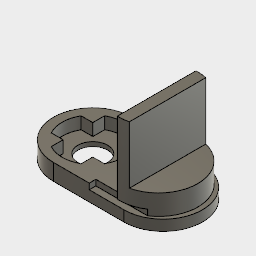
servo_bracket_elbow_1 (Autodesk Fusion 360 design; units mm, degrees)
Autodesk Fusion 360 part; units mm, degrees
sketch "スケッチ1" plane through (0, 0, 0) normal (0, 1, 0) x (1, 0, 0)
  circle A0 centre (0, 0) radius 7.15
  line L0 (0, 0) -> (0, 7.15)
  line L1 (0, 0) -> (0, -7.15)
  line L2 (0, 7.15) -> (0, -7.15)
  line L3 (0, -7.15) -> (12.8, -7.15)
  line L4 (12.8, -7.15) -> (12.8, 7.15)
  line L5 (12.8, 7.15) -> (0, 7.15)
  circle A1 centre (12.8, 0) radius 7.15
  circle A2 centre (0, 0) radius 5.55
  circle A3 centre (0, 0) radius 2.7
  line L6 (2.7, 2.7) -> (-2.7, 2.7) construction
  line L7 (-2.7, 2.7) -> (-2.7, -2.7) construction
  line L8 (-2.7, -2.7) -> (2.7, -2.7) construction
  line L9 (2.7, -2.7) -> (2.7, 2.7) construction
  line L10 (2.7, 2.7) -> (-2.7, -2.7) construction
  line L11 (-2.7, 2.7) -> (2.7, -2.7) construction
  line L12 (-2.7, 2.7) -> (-4.849, 2.7)
  line L13 (-2.7, 2.7) -> (-2.7, 4.849)
  line L14 (-2.7, -2.7) -> (-4.849, -2.7)
  line L15 (-2.7, -2.7) -> (-2.7, -4.849)
  line L16 (2.7, -2.7) -> (2.7, -4.849)
  line L17 (2.7, -2.7) -> (4.849, -2.7)
  line L18 (2.7, 2.7) -> (4.849, 2.7)
  line L19 (2.7, 2.7) -> (2.7, 4.849)
  dimension "d1" = 14.3
  dimension "d2" = 12.8
  dimension "d5" = 11.1
  dimension "d6" = 5.4
  dimension "d7" = 5.4
  dimension "d8" = 5.4
  constraint coincident A0
  constraint vertical L0
  constraint parallel L0 L1
  constraint perpendicular L2 L3
  constraint parallel L2 L4
  constraint parallel L3 L5
  constraint midpoint L4
  constraint coincident A1
  constraint concentric A2 A3
  constraint perpendicular L6 L7
  constraint parallel L6 L8
  constraint parallel L7 L9
  constraint horizontal L6
  constraint coincident L10
  constraint coincident L11
  constraint coincident A2
  constraint perpendicular L7 L12
  constraint perpendicular L12 L13
  constraint perpendicular L13 L14
  constraint perpendicular L14 L15
  constraint perpendicular L8 L16
  constraint perpendicular L16 L17
  constraint perpendicular L9 L18
  constraint perpendicular L18 L19
  measures "d1" diameter of A0
  measures "d5" diameter of A2
  measures "d6" diameter of A3
extrude "押し出し1" add sketch "スケッチ1" against normal blind 3
extrude "押し出し2" cut sketch "スケッチ1" against normal blind 2.2 contours L0 L1 L2 A2 A3 L16 L17 L18 L19 | L0 L1 L2 A2 A3 L12 L13 L14 L15
extrude "押し出し3" cut sketch "スケッチ1" against normal blind 6 contours L0 L1 L2 A3 | L0 L1 L2 A3
sketch "スケッチ2" plane through (0, 0, 0) normal (0, 1, 0) x (1, 0, 0)
  line L0 (12.8, 0) -> (11.95, 0)
  circle A0 centre (11.95, 0) radius 7.15
  line L1 (12.8, 0) -> (11.6, 0)
  line L2 (0, 7.15) -> (12.8, 7.15)
  line L3 (11.6, 0) -> (11.6, 7.15)
  line L4 (12.8, -7.15) -> (0, -7.15)
  line L5 (11.6, 0) -> (11.6, -7.1414)
  line L6 (11.6, 0) -> (13.6, 0)
  line L7 (13.6, 0) -> (13.6, 6.957)
  line L8 (13.6, 0) -> (13.6, -6.957)
  dimension "d13" = 0.85
  dimension "d14" = 14.3
  dimension "d15" = 1.2
  dimension "d16" = 2
  constraint coincident L2
  constraint coincident A0
  constraint perpendicular L4 L5
  constraint perpendicular L6 L7
  constraint perpendicular L6 L8
  measures "d14" diameter of A0
extrude "押し出し4" add sketch "スケッチ2" along normal blind 2.65 contours A0 L7 L8
extrude "押し出し5" add sketch "スケッチ2" along normal blind 13.5 contours L0 A0 L1 L5 L6 L8 | L0 A0 L1 L3 L6 L7
sketch "スケッチ3" plane through (0, 0, 7.15) normal (0, 0, 1) x (1, 0, 0)
  line L0 (11.95, 0) -> (0, 0)
  line L1 (0, 0) -> (0, -3)
  line L2 (0, -3) -> (12.8, -3)
  line L3 (12.8, -3) -> (12.8, 0)
  line L4 (12.8, 0) -> (11.95, 0)
  line L5 (0, -3) -> (6.5, -3)
  line L6 (6.5, -3) -> (6.5, -1.05)
  line L7 (6.5, -1.05) -> (0, -1.05)
  line L8 (0, -1.05) -> (0, -3)
  line L9 (6.5, -1.05) -> (16.5, -1.05)
  line L10 (16.5, -1.05) -> (16.5, 0.4)
  line L11 (16.5, 0.4) -> (6.5, 0.4)
  line L12 (6.5, 0.4) -> (6.5, -1.05)
  dimension "d21" = 6.5
  dimension "d22" = 1.95
  dimension "d23" = 10
  dimension "d24" = 1.45
  constraint horizontal L5
  constraint vertical L6
  constraint horizontal L7
  constraint vertical L8
  constraint horizontal L9
  constraint vertical L10
  constraint horizontal L11
  constraint vertical L12
extrude "押し出し6" cut sketch "スケッチ3" against normal blind 1.2 contours L0 L3 L4 L9 L12 | L0 L3 L4 L9 L10 L11 L12
sketch "スケッチ4" plane through (0, 0, -7.15) normal (0, 0, -1) x (-1, 0, 0)
  line L0 (-11.95, 0) -> (-12.8, 0)
  line L1 (-12.8, 0) -> (-12.8, -3)
  line L2 (-12.8, -3) -> (0, -3)
  line L3 (0, -3) -> (0, 0)
  line L4 (0, 0) -> (-11.95, 0)
  line L5 (0, -3) -> (-6.5, -3)
  line L6 (-6.5, -3) -> (-6.5, -1.05)
  line L7 (-6.5, -1.05) -> (0, -1.05)
  line L8 (0, -1.05) -> (0, -3)
  line L9 (-6.5, -1.05) -> (-16.5, -1.05)
  line L10 (-16.5, -1.05) -> (-16.5, 0.4)
  line L11 (-16.5, 0.4) -> (-6.5, 0.4)
  line L12 (-6.5, 0.4) -> (-6.5, -1.05)
  dimension "d27" = 6.5
  dimension "d28" = 1.95
  constraint horizontal L5
  constraint vertical L6
  constraint horizontal L7
  constraint vertical L8
  constraint horizontal L9
  constraint vertical L10
  constraint horizontal L11
  constraint vertical L12
extrude "押し出し7" cut sketch "スケッチ4" against normal blind 1.2 contours L0 L1 L4 L9 L12 | L0 L1 L4 L9 L10 L11 L12
extrude "押し出し8" cut 1 faces at (19.5158, 0, -1.3712) along direction (0, -1, 0) blind 1.05
extrude "押し出し9" add 2 faces at (11.9033, 0.4, 6.7398) (11.9033, 0.4, -6.7398) along direction (0, -1, 0) blind 0.4
extrude "押し出し10" cut 1 faces at (12.7143, 13.5, -2.319) along direction (0, -1, 0) blind 0.4
